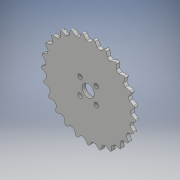
# Autodesk Inventor part: kolo 25  8,3 mm 147 dg 4,3 mm
Saved by Autodesk Inventor 2017 (Build 210142000, 142)
## iProperties
Created: 2019-08-27
Part Number: kolo 25  8,3 mm 147 dg 4,3 mm
Material: Ogólny
Document SubType Name: Modeling
Designer: patry
Density: 1 g/cm^3
Appearance: Domyślna
Author: patry
Autodesk Inventor part; units mm, degrees
ref_plane "YZ Plane" through (0, 0, 0) normal (1, 0, 0) x (0, 1, 0)
ref_plane "XZ Plane" through (0, 0, 0) normal (0, 1, 0) x (-1, 0, 0)
ref_plane "XY Plane" through (0, 0, 0) normal (0, 0, 1) x (1, 0, 0)
sketch "Szkic2" plane through (0, 0, 0) normal (0, 1, 0) x (-1, 0, 0)
  line L0 (0, 0) -> (-3.962, -31.3625) construction
  line L1 (0, 0) -> (3.962, -31.3625) construction
  line L2 (3.962, -31.3625) -> (-3.962, -31.3625) construction
  line L3 (0, 0) -> (0, -151) construction
  circle A0 centre (0, 0) radius 31.6117 construction
  line L4 (0, -35.6625) -> (2.7059, -31.4957) construction
  line L5 (0, -35.6625) -> (-2.7059, -31.4957) construction
  circle A1 centre (0, -33.9051) radius 0.9571 construction
  line L6 (2.7059, -31.4957) -> (0.8027, -34.4264)
  line L7 (-2.7059, -31.4957) -> (-0.8027, -34.4264)
  arc A2 (-0.8027, -34.4264) -> (0.8027, -34.4264) centre (0, -33.9051) ccw
  line L8 (-2.7059, -31.4957) -> (5.2118, -31.1791) construction
  arc A3 (2.7059, -31.4957) -> (5.2118, -31.1791) centre (0, 0) ccw
  line L9 (8.8689, -34.5421) -> (5.2118, -31.1791) construction
  line L10 (5.2118, -31.1791) -> (7.784, -33.5445)
  arc A4 (7.784, -33.5445) -> (9.339, -33.1452) centre (8.4319, -32.8399) ccw
  line L11 (10.4536, -29.8333) -> (9.339, -33.1452)
  arc A5 (10.4536, -29.8333) -> (12.802, -28.9035) centre (0, 0) ccw
  line L12 (17.1805, -31.2513) -> (12.802, -28.9035) construction
  line L13 (12.802, -28.9035) -> (15.8816, -30.5548)
  arc A6 (15.8816, -30.5548) -> (17.2885, -29.7814) centre (16.3339, -29.7113) ccw
  line L14 (17.5444, -26.2963) -> (17.2885, -29.7814)
  arc A7 (17.5444, -26.2963) -> (19.5878, -24.8117) centre (0, 0) ccw
  line L15 (24.4126, -25.9968) -> (19.5878, -24.8117) construction
  line L16 (19.5878, -24.8117) -> (22.9813, -25.6453)
  arc A8 (22.9813, -25.6453) -> (24.1516, -24.5463) centre (23.2096, -24.7158) ccw
  line L17 (23.5328, -21.107) -> (24.1516, -24.5463)
  arc A9 (23.5328, -21.107) -> (25.1428, -19.1609) centre (0, 0) ccw
  line L18 (30.1108, -19.1089) -> (25.1428, -19.1609) construction
  line L19 (25.1428, -19.1609) -> (28.6371, -19.1243)
  arc A10 (28.6371, -19.1243) -> (29.4973, -17.7688) centre (28.627, -18.1673) ccw
  line L20 (28.0426, -14.5916) -> (29.4973, -17.7688)
  arc A11 (28.0426, -14.5916) -> (29.118, -12.3062) centre (0, 0) ccw
  line L21 (33.917, -11.0203) -> (29.118, -12.3062) construction
  line L22 (29.118, -12.3062) -> (32.4934, -11.4018)
  arc A12 (32.4934, -11.4018) -> (32.9895, -9.8749) centre (32.2457, -10.4773) ccw
  line L23 (30.7904, -7.1592) -> (32.9895, -9.8749)
  arc A13 (30.7904, -7.1592) -> (31.2636, -4.6782) centre (0, 0) ccw
  line L24 (35.5921, -2.2393) -> (31.2636, -4.6782) construction
  line L25 (31.2636, -4.6782) -> (34.3081, -2.9628)
  arc A14 (34.3081, -2.9628) -> (34.4089, -1.3605) centre (33.8382, -2.1289) ccw
  line L26 (31.6035, 0.723) -> (34.4089, -1.3605)
  arc A15 (31.6035, 0.723) -> (31.4449, 3.2437) centre (0, 0) ccw
  line L27 (35.0308, 6.6825) -> (31.4449, 3.2437) construction
  line L28 (31.4449, 3.2437) -> (33.967, 5.6624)
  arc A16 (33.967, 5.6624) -> (33.6662, 7.2394) centre (33.3046, 6.3532) ccw
  line L29 (30.4308, 8.5597) -> (33.6662, 7.2394)
  arc A17 (30.4308, 8.5597) -> (29.6503, 10.9618) centre (0, 0) ccw
  line L30 (32.2684, 15.1843) -> (29.6503, 10.9618) construction
  line L31 (29.6503, 10.9618) -> (31.4917, 13.9317)
  arc A18 (31.4917, 13.9317) -> (30.8082, 15.3844) centre (30.6783, 14.4361) ccw
  line L32 (27.346, 15.8586) -> (30.8082, 15.3844)
  arc A19 (27.346, 15.8586) -> (25.9927, 17.9912) centre (0, 0) ccw
  line L33 (27.4784, 22.7321) -> (25.9927, 17.9912) construction
  line L34 (25.9927, 17.9912) -> (27.0377, 21.3257)
  arc A20 (27.0377, 21.3257) -> (26.0143, 22.5627) centre (26.1243, 21.6119) ccw
  line L35 (22.543, 22.1611) -> (26.0143, 22.5627)
  arc A21 (22.543, 22.1611) -> (20.7018, 23.8901) centre (0, 0) ccw
  line L36 (20.9619, 28.8515) -> (20.7018, 23.8901) construction
  line L37 (20.7018, 23.8901) -> (20.8847, 27.3797)
  arc A22 (20.8847, 27.3797) -> (19.5859, 28.3234) centre (19.9289, 27.4298) ccw
  line L38 (16.3236, 27.0711) -> (19.5859, 28.3234)
  arc A23 (16.3236, 27.0711) -> (14.1102, 28.2878) centre (0, 0) ccw
  line L39 (13.1282, 33.1581) -> (14.1102, 28.2878) construction
  line L40 (14.1102, 28.2878) -> (13.4195, 31.7134)
  arc A24 (13.4195, 31.7134) -> (11.9269, 32.3043) centre (12.4813, 31.5242) ccw
  line L41 (9.0784, 30.2801) -> (11.9269, 32.3043)
  arc A25 (9.0784, 30.2801) -> (6.632, 30.9082) centre (0, 0) ccw
  line L42 (4.4697, 35.3813) -> (6.632, 30.9082) construction
  line L43 (6.632, 30.9082) -> (5.1112, 34.0543)
  arc A26 (5.1112, 34.0543) -> (3.5184, 34.2555) centre (4.2494, 33.6378) ccw
  line L44 (1.2629, 31.5865) -> (3.5184, 34.2555)
  arc A27 (1.2629, 31.5865) -> (-1.2629, 31.5865) centre (0, 0) ccw
  line L45 (-4.4697, 35.3813) -> (-1.2629, 31.5865) construction
  line L46 (-1.2629, 31.5865) -> (-3.5184, 34.2555)
  arc A28 (-3.5184, 34.2555) -> (-5.1112, 34.0543) centre (-4.2494, 33.6378) ccw
  line L47 (-6.632, 30.9082) -> (-5.1112, 34.0543)
  arc A29 (-6.632, 30.9082) -> (-9.0784, 30.2801) centre (0, 0) ccw
  line L48 (-13.1282, 33.1581) -> (-9.0784, 30.2801) construction
  line L49 (-9.0784, 30.2801) -> (-11.9269, 32.3043)
  arc A30 (-11.9269, 32.3043) -> (-13.4195, 31.7134) centre (-12.4813, 31.5242) ccw
  line L50 (-14.1102, 28.2878) -> (-13.4195, 31.7134)
  arc A31 (-14.1102, 28.2878) -> (-16.3236, 27.0711) centre (0, 0) ccw
  line L51 (-20.9619, 28.8515) -> (-16.3236, 27.0711) construction
  line L52 (-16.3236, 27.0711) -> (-19.5859, 28.3234)
  arc A32 (-19.5859, 28.3234) -> (-20.8847, 27.3797) centre (-19.9289, 27.4298) ccw
  line L53 (-20.7018, 23.8901) -> (-20.8847, 27.3797)
  arc A33 (-20.7018, 23.8901) -> (-22.543, 22.1611) centre (0, 0) ccw
  line L54 (-27.4784, 22.7321) -> (-22.543, 22.1611) construction
  line L55 (-22.543, 22.1611) -> (-26.0143, 22.5627)
  arc A34 (-26.0143, 22.5627) -> (-27.0377, 21.3257) centre (-26.1243, 21.6119) ccw
  line L56 (-25.9927, 17.9912) -> (-27.0377, 21.3257)
  arc A35 (-25.9927, 17.9912) -> (-27.346, 15.8586) centre (0, 0) ccw
  line L57 (-32.2684, 15.1843) -> (-27.346, 15.8586) construction
  line L58 (-27.346, 15.8586) -> (-30.8082, 15.3844)
  arc A36 (-30.8082, 15.3844) -> (-31.4917, 13.9317) centre (-30.6783, 14.4361) ccw
  line L59 (-29.6503, 10.9618) -> (-31.4917, 13.9317)
  arc A37 (-29.6503, 10.9618) -> (-30.4308, 8.5597) centre (0, 0) ccw
  line L60 (-35.0308, 6.6825) -> (-30.4308, 8.5597) construction
  line L61 (-30.4308, 8.5597) -> (-33.6662, 7.2394)
  arc A38 (-33.6662, 7.2394) -> (-33.967, 5.6624) centre (-33.3046, 6.3532) ccw
  line L62 (-31.4449, 3.2437) -> (-33.967, 5.6624)
  arc A39 (-31.4449, 3.2437) -> (-31.6035, 0.723) centre (0, 0) ccw
  line L63 (-35.5921, -2.2393) -> (-31.6035, 0.723) construction
  line L64 (-31.6035, 0.723) -> (-34.4089, -1.3605)
  arc A40 (-34.4089, -1.3605) -> (-34.3081, -2.9628) centre (-33.8382, -2.1289) ccw
  line L65 (-31.2636, -4.6782) -> (-34.3081, -2.9628)
  arc A41 (-31.2636, -4.6782) -> (-30.7904, -7.1592) centre (0, 0) ccw
  line L66 (-33.917, -11.0203) -> (-30.7904, -7.1592) construction
  line L67 (-30.7904, -7.1592) -> (-32.9895, -9.8749)
  arc A42 (-32.9895, -9.8749) -> (-32.4934, -11.4018) centre (-32.2457, -10.4773) ccw
  line L68 (-29.118, -12.3062) -> (-32.4934, -11.4018)
  arc A43 (-29.118, -12.3062) -> (-28.0426, -14.5916) centre (0, 0) ccw
  line L69 (-30.1108, -19.1089) -> (-28.0426, -14.5916) construction
  line L70 (-28.0426, -14.5916) -> (-29.4973, -17.7688)
  arc A44 (-29.4973, -17.7688) -> (-28.6371, -19.1243) centre (-28.627, -18.1673) ccw
  line L71 (-25.1428, -19.1609) -> (-28.6371, -19.1243)
  arc A45 (-25.1428, -19.1609) -> (-23.5328, -21.107) centre (0, 0) ccw
  line L72 (-24.4126, -25.9968) -> (-23.5328, -21.107) construction
  line L73 (-23.5328, -21.107) -> (-24.1516, -24.5463)
  arc A46 (-24.1516, -24.5463) -> (-22.9813, -25.6453) centre (-23.2096, -24.7158) ccw
  line L74 (-19.5878, -24.8117) -> (-22.9813, -25.6453)
  arc A47 (-19.5878, -24.8117) -> (-17.5444, -26.2963) centre (0, 0) ccw
  line L75 (-17.1805, -31.2513) -> (-17.5444, -26.2963) construction
  line L76 (-17.5444, -26.2963) -> (-17.2885, -29.7814)
  arc A48 (-17.2885, -29.7814) -> (-15.8816, -30.5548) centre (-16.3339, -29.7113) ccw
  line L77 (-12.802, -28.9035) -> (-15.8816, -30.5548)
  arc A49 (-12.802, -28.9035) -> (-10.4536, -29.8333) centre (0, 0) ccw
  line L78 (-8.8689, -34.5421) -> (-10.4536, -29.8333) construction
  line L79 (-10.4536, -29.8333) -> (-9.339, -33.1452)
  arc A50 (-9.339, -33.1452) -> (-7.784, -33.5445) centre (-8.4319, -32.8399) ccw
  line L80 (-5.2118, -31.1791) -> (-7.784, -33.5445)
  arc A51 (-5.2118, -31.1791) -> (-2.7059, -31.4957) centre (0, 0) ccw
  dimension "d19" = 7.924
  dimension "d20" = 3.962
  dimension "d21" = 14.4
  dimension "d22" = 4.3
  dimension "d23" = 147
  dimension "d24" = 147
  dimension "d26" = 7.924
  dimension "d44" = 1.7573
  constraints: 162 end point, 106 point on circle, 52 centre point, 28 point on line, 2 coincident, 2 tangent, 1 concentric, 1 equal length, 1 vertical, 2 other
  measures "d19" distance of L1.end L0.end
  measures "d20" distance from line of L1.end L3
  measures "d21" angle of L1 L0
  measures "d22" distance from line of L2 L4.start
  measures "d23" angle of L3 L4
  measures "d24" angle of L3 L5
  measures "d26" distance of L5.end L8.end
  measures "d44" distance of L4.start point (0, -33.905)
sketch "Szkic3" plane through (0, 0, 0) normal (0, 1, 0) x (-1, 0, 0)
  circle A0 centre (0, 0) radius 8.5 construction
  line L0 (-6.0104, 6.0104) -> (6.0104, 6.0104) construction
  line L1 (6.0104, 6.0104) -> (6.0104, -6.0104) construction
  line L2 (6.0104, -6.0104) -> (-6.0104, -6.0104) construction
  line L3 (-6.0104, -6.0104) -> (-6.0104, 6.0104) construction
  line L4 (-6.0104, 6.0104) -> (6.0104, -6.0104) construction
  line L5 (6.0104, 6.0104) -> (-6.0104, -6.0104) construction
  dimension "d37" = 17
  constraints: 12 end point, 5 coincident, 2 midpoint, 2 parallel, 2 perpendicular, 1 horizontal, 3 other
extrude "Wyciągnięcie proste2" add sketch "Szkic2" along normal blind 2.5
hole "Otwór1" at (-6.0104, 0, -6.0104) at (6.0104, 0, -6.0104) at (6.0104, 0, 6.0104) at (-6.0104, 0, 6.0104) direction (0, 1, 0) diameter 3.3 end through all
sketch "Szkic4" plane through (0, 0, 0) normal (0, -1, 0) x (1, 0, 0)
  point P0 (0, 0)
  point P1 (0, 0)
  constraints: 1 coincident
hole "Otwór2" at (0, 0, 0) direction (0, 1, 0) diameter 9 end through all
equation "\"d19\" = dl_przeskoku"
equation "\"d20\" = 0.5 * d19"
equation "\"d23\" = kat_zeba"
equation "\"d24\" = kat_zeba"
equation "\"d26\" = dl_przeskoku"
equation "\"kat\" = 360deg"
equation "\"kat_zeba\" = 147deg"
equation "\"wys_zeba\" = 5"
equation "\"odl_osi_zeba\" = 2.366"
equation "\"dl_ogniwa\" = 8.3"
equation "\"dl_przeskoku\" = 7.924"
